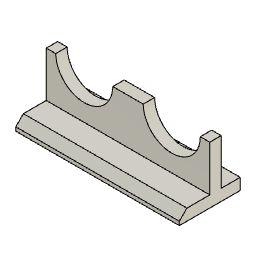
ピンバイス置き (Autodesk Fusion 360 design; units mm, degrees)
Autodesk Fusion 360 part; units mm, degrees
sketch "スケッチ1" plane through (0, 0, 0) normal (0, 1, 0) x (1, 0, 0)
  line L0 (-7.4996, -9.9227) -> (-10, -9.9227)
  line L1 (-10, -9.9227) -> (-10, 0)
  line L2 (-10, 0) -> (-10, 5)
  line L3 (-10, 5) -> (10, 5)
  line L4 (10, 5) -> (10, -10)
  line L5 (10, -10) -> (7.5, -10)
  arc A0 (7.5, -10) -> (-7.4996, -9.9227) centre (0, -10) ccw
  dimension "d1" = 15
  constraint horizontal L0
  constraint perpendicular L0 L1
  constraint perpendicular L0 L2
  constraint perpendicular L2 L3
  constraint perpendicular L3 L4
  constraint perpendicular L4 L5
  measures "d1" diameter of A0
extrude "押し出し1" add sketch "スケッチ1" along normal blind 3 makes body 1
sketch "スケッチ2" plane through (0, 0, 0) normal (0, -1, 0) x (1, 0, 0)
  line L0 (10, 10) -> (7.5, 10)
  arc A0 (-7.4996, 9.9227) -> (7.5, 10) centre (0, 10) ccw
  line L1 (-7.4996, 9.9227) -> (-10, 9.9227)
  line L2 (-10, 9.9227) -> (-10, -5)
  line L3 (-10, -5) -> (10, -5)
  line L4 (10, -5) -> (10, 10)
  line L5 (-10, -2) -> (10, -2)
  constraint coincident L2 L5.start
  constraint coincident L4 L5.end
  constraint perpendicular L4 L5
extrude "押し出し2" add sketch "スケッチ2" along normal blind 8 and the other way blind 8 contours L2 L3 L4 L5 bodies 1
chamfer "面取り1" distance 2 angle 45 1 edges at (0, -8, -2) on bodies 1
copy_body "ボディのコピーと貼り付け1" bodies 1 makes body 2
move_body "移動1" bodies 2 to x (1, 0, 0) y (0, 1, 0) z (0, 0, 1) at (20, 0, 0)
combine "結合1" operation add target body 1 tool bodies 2
delete_face "面を削除1" 1 faces at (10, 1, 9.9485) on bodies 1
ref_plane "作業平面1" through (10, 0, 2.4614) normal (-1, 0, 0) x (0, 0, 1)
split "分割2" by plane through (10, 0, 2.4614) normal (-1, 0, 0) bodies 1 makes body 3 at (-3.3333, -2.6667, -5)
move_body "移動2" bodies 1 to x (1, 0, 0) y (0, 1, 0) z (0, 0, 1) at (3, 0, 0)
move_face "面を移動1" by (-4, 0, 0) 1 faces at (13, 0, -4) on bodies 1
combine "結合2" operation add target body 3 tool bodies 1
